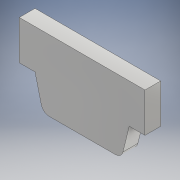
# Autodesk Inventor part: RightAngleLED
Saved by Autodesk Inventor 2017 (Build 210142000, 142)
## iProperties
Created: 2018-08-14
Part Number: RightAngleLED
Material: Generic
Document SubType Name: Modeling
Designer: intelsath
Density: 1 g/cm^3
Appearance: Default
Author: intelsath
Autodesk Inventor part; units mm, degrees
ref_plane "YZ Plane" through (0, 0, 0) normal (1, 0, 0) x (0, 1, 0)
ref_plane "XZ Plane" through (0, 0, 0) normal (0, 1, 0) x (-1, 0, 0)
ref_plane "XY Plane" through (0, 0, 0) normal (0, 0, 1) x (1, 0, 0)
sketch "Sketch1" plane through (0, 0, 0) normal (0, 1, 0) x (-1, 0, 0)
  line L0 (0.8, 0.25) -> (-0.8, 0.25)
  line L1 (-0.8, 0.25) -> (-0.8, -0.25)
  line L2 (-0.8, -0.25) -> (0.8, -0.25)
  line L3 (0.8, -0.25) -> (0.8, 0.25)
  line L4 (0.8, 0.25) -> (-0.8, -0.25) construction
  line L5 (-0.8, 0.25) -> (0.8, -0.25) construction
  point P0 (0, 0)
  dimension "d0" = 0.5
  dimension "d1" = 1.6
  constraints: 12 end point, 2 midpoint, 2 parallel, 1 horizontal, 1 perpendicular
  measures "d0" distance of L0.end L1.end
  measures "d1" distance of L1.end L2.end
extrude "Extrusion1" add sketch "Sketch1" along normal blind 0.2
sketch "Sketch2" plane through (0, 0, 0) normal (0, 1, 0) x (-1, 0, 0)
  line L0 (-0.8, -0.25) -> (0.8, -0.25) projected
  line L1 (0.6, -0.25) -> (0.5189, -0.5743)
  line L2 (0.4219, -0.65) -> (-0.4219, -0.65)
  line L3 (-0.5189, -0.5743) -> (-0.6, -0.25)
  line L4 (0.8, 0.25) -> (-0.8, 0.25) projected
  line L5 (0.6, -0.25) -> (-0.6, -0.25)
  arc A0 (0.4219, -0.65) -> (0.5189, -0.5743) centre (0.4219, -0.55) ccw
  arc A1 (-0.5189, -0.5743) -> (-0.4219, -0.65) centre (-0.4219, -0.55) ccw
  point P0 (0, 0)
  point P1 (0.5, -0.65)
  point P2 (-0.5, -0.65)
  point P3 (0, -0.25)
  dimension "d4" = 0.9
  dimension "d6" = 1.2
  dimension "d7" = 1
  dimension "d8" = 0.1
  constraints: 8 end point, 6 point on line, 4 point on circle, 4 tangent, 2 centre point, 2 midpoint, 1 collinear, 1 equal length, 1 equal radius, 1 horizontal, 1 vertical alignment
  measures "d4" distance between parallel lines of L4 L2
  measures "d6" distance of L1.start L3.end
  measures "d7" distance of point (0.5, -0.65) point (-0.5, -0.65)
  measures "d8" radius of A0
extrude "Extrusion2" add sketch "Sketch2" along normal blind 0.19
body "Solid1"
